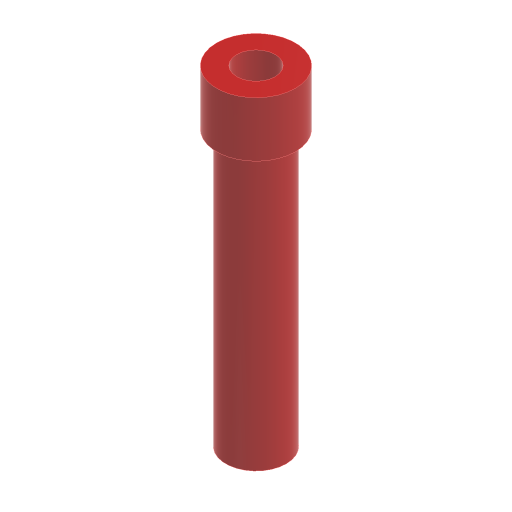
# Autodesk Inventor part: Arduino-cz1
Saved by Autodesk Inventor 2024.3 (Build 283343000, 343)
## iProperties
Created: 2025-06-24
Part Number: Arduino-cz1
Material: PET Plastic
Document SubType Name: Modeling
Designer: MPA
Density: 1.541 g/cm^3
Appearance: Red
Author: MPA
## iProperties of the stored document Arduino-cz1_3DPrint.ipt
Created: 2025-06-24
Part Number: Arduino-cz1_3DPrint
Material: Generic
Document SubType Name: Modeling
Designer: MPA
Density: 1 g/cm^3
Appearance: Default
Author: MPA
Autodesk Inventor part; units mm, degrees
ref_plane "YZ Plane" through (0, 0, 0) normal (1, 0, 0) x (0, 1, 0)
ref_plane "XZ Plane" through (0, 0, 0) normal (0, 1, 0) x (-1, 0, 0)
ref_plane "XY Plane" through (0, 0, 0) normal (0, 0, 1) x (1, 0, 0)
sketch "Sketch1" plane through (0, 0, 0) normal (0, 1, 0) x (-1, 0, 0)
  circle A0 centre (0, 0) radius 1.65
  circle A1 centre (0, 0) radius 1.05
  dimension "d0" = 3.3
  dimension "d1" = 2.1
  constraints: 2 centre point, 2 coincident
  measures "d0" diameter of A0
  measures "d1" diameter of A1
extrude "Extrusion1" add sketch "Sketch1" along normal blind 15
sketch "Sketch2" plane through (0, 15, 0) normal (0, 1, 0) x (1, 0, 0)
  circle A0 centre (0, 0) radius 1.65 projected
  circle A1 centre (0, 0) radius 1.05 projected
  circle A2 centre (0, 0) radius 2.15
  dimension "d4" = 0.5
  constraints: 1 centre point
  measures "d4" radial gap between concentric circles of A0 A2
extrude "Extrusion2" add sketch "Sketch2" along normal blind 3 contours A0 | A2
body "Solid1"
